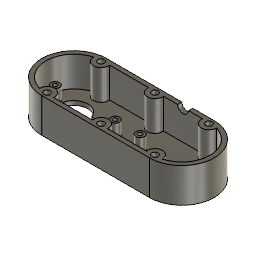
robosoc_motor_case_with_hole (Autodesk Fusion 360 design; units mm, degrees)
part number: 2025-12-10-15-49-31-313
Autodesk Fusion 360 part; units mm, degrees
sketch "Sketch1" plane through (0, 0, 0) normal (0, 0, 1) x (1, 0, 0)
  line L0 (15, 0) -> (65, 0)
  line L1 (65, 30) -> (15, 30)
  arc A0 (15, 30) -> (0, 15) centre (15, 15) ccw
  arc A1 (0, 15) -> (15, 0) centre (15, 15) ccw
  arc A2 (80, 15) -> (65, 30) centre (65, 15) ccw
  arc A3 (65, 0) -> (80, 15) centre (65, 15) ccw
  line L2 (15, 15) -> (65, 15) construction
  line L3 (15, 15) -> (15, 27.5) construction
  line L4 (65, 15) -> (65, 27.5) construction
  line L5 (15, 27.5) -> (40, 27.5) construction
  circle A4 centre (15, 27.5) radius 1.5
  circle A5 centre (40, 27.5) radius 1.5
  circle A6 centre (65, 27.5) radius 1.5
  circle A7 centre (15, 2.5) radius 1.5
  circle A8 centre (40, 2.5) radius 1.5
  circle A9 centre (65, 2.5) radius 1.5
  point P0 (80, 0)
  point P1 (0, 30)
  dimension "d1" = 80
  dimension "d2" = 30
  dimension "d3" = 15
  dimension "d4" = 15
  dimension "d5" = 15
  dimension "d6" = 15
  dimension "d7" = 12.5
  dimension "d8" = 12.5
  dimension "d9" = 25
  dimension "d11" = 3
  dimension "d12" = 3
  dimension "d13" = 3
  constraint horizontal L0
  constraint horizontal L1
  constraint coincident P1 L1
  constraint tangent L1 A0
  constraint coincident origin L0
  constraint tangent L0 A1
  constraint coincident A0.end A1.start
  constraint tangent L1 A2
  constraint coincident P0 L0
  constraint tangent L0 A3
  constraint coincident A2.start A3.end
  constraint coincident A0.centre A1.centre
  constraint coincident A2.centre A3.centre
  constraint perpendicular L1 L3
  constraint perpendicular L2 L4
  constraint perpendicular L3 L5
  constraint coincident L3.end L5.start
  constraint coincident L5.end A5.centre
  constraint coincident L4.end A6.centre
  constraint symmetric L2 A4 A7
  constraint symmetric L2 A5 A8
  constraint symmetric L2 A6 A9
  measures "d1" distance of origin P0
  measures "d2" distance of origin P1
  measures "d3" radius of A0
  measures "d4" radius of A1
  measures "d5" radius of A2
  measures "d6" radius of A3
  measures "d7" distance of A0.centre L3.end
  measures "d8" distance of A2.centre L4.end
  measures "d9" distance of L3.end L5.end
  measures "d11" diameter of A4
  measures "d12" diameter of A5
  measures "d13" diameter of A6
extrude "Extrude4" add sketch "Sketch1" along normal blind 2 contours A4 | A5 | A6 | A7 | A8 | A9 makes body 1 at (63.9526, 26.4262, 1.3333) makes body 2 at (41.4981, 2.4252, 1.3333) makes body 3 at (63.9526, 1.4262, 1.3333) makes body 4 at (38.9526, 26.4262, 1.3333) makes body 5 at (16.4981, 27.4252, 1.3333) makes body 6 at (16.4981, 2.4252, 1.3333)
extrude "Extrude1" add sketch "Sketch1" along normal blind 16 separate body makes body 7
shell "Shell1" thickness 2 removed faces 1 at (23.6999, 18.8266, 16) on bodies 7
sketch "Sketch2" plane through (0, 0, 2) normal (0, 0, 1) x (-1, 0, 0)
  arc A0 (-68.4999, -2.48) -> (-61.5359, -2) centre (-65, -2.5) ccw
  arc A1 (-68.4999, -2.48) -> (-68.4999, -27.52) centre (-65, -15) ccw
  arc A2 (-61.5359, -28) -> (-68.4999, -27.52) centre (-65, -27.5) ccw
  line L0 (-61.5359, -28) -> (-43.4641, -28)
  arc A3 (-36.5359, -28) -> (-43.4641, -28) centre (-40, -27.5) ccw
  line L1 (-36.5359, -28) -> (-18.4641, -28)
  arc A4 (-11.5001, -27.52) -> (-18.4641, -28) centre (-15, -27.5) ccw
  arc A5 (-11.5001, -27.52) -> (-11.5001, -2.48) centre (-15, -15) ccw
  arc A6 (-18.4641, -2) -> (-11.5001, -2.48) centre (-15, -2.5) ccw
  line L2 (-18.4641, -2) -> (-36.5359, -2)
  arc A7 (-43.4641, -2) -> (-36.5359, -2) centre (-40, -2.5) ccw
  line L3 (-43.4641, -2) -> (-61.5359, -2)
  line L4 (-15, -2.5) -> (-15, -27.5) construction
  arc A8 (-20.7264, -12.142) -> (-20.9934, -17.2449) centre (-21.0208, -14.6851) ccw
  arc A9 (-20.9934, -17.2449) -> (-20.7264, -12.142) centre (-15, -15) ccw
  arc A10 (-58.9129, -12.4127) -> (-58.8845, -17.522) centre (-64.7667, -15) ccw
  arc A11 (-58.8845, -17.522) -> (-58.9129, -12.4127) centre (-58.7336, -14.9664) ccw
  line L5 (-15, -15) -> (-34.1, -15) construction
  line L6 (-15, -15) -> (-6.3, -15) construction
  line L7 (-64.7667, -15) -> (-45.6667, -15) construction
  line L8 (-64.7667, -15) -> (-73.4667, -15) construction
  circle A12 centre (-6.3, -15) radius 1
  circle A13 centre (-34.1, -15) radius 1
  circle A14 centre (-73.4667, -15) radius 1
  circle A15 centre (-45.6667, -15) radius 1
  circle A16 centre (-34.1, -15) radius 2
  circle A17 centre (-6.3, -15) radius 2
  circle A18 centre (-45.6667, -15) radius 2
  circle A19 centre (-73.4667, -15) radius 2
  dimension "d17" = 12.8
  dimension "d18" = 12.8
  dimension "d19" = 5.12
  dimension "d20" = 5.12
  dimension "d22" = 19.1
  dimension "d23" = 8.7
  dimension "d24" = 19.1
  dimension "d25" = 8.7
  dimension "d26" = 2
  dimension "d27" = 2
  dimension "d29" = 2
  dimension "d31" = 2
  dimension "d32" = 1
  dimension "d33" = 1
  dimension "d34" = 1
  dimension "d35" = 1
  constraint coincident A6.centre L4.start
  constraint coincident A4.centre L4.end
  constraint concentric A5 A9
  constraint coincident A5.centre A9.centre
  constraint perpendicular L4 L5
  constraint perpendicular L4 L6
  constraint coincident A10.centre L7.start
  constraint parallel L1 L7
  constraint parallel L7 L8
  constraint coincident L6.end A12.centre
  constraint coincident L5.end A13.centre
  constraint coincident L8.end A14.centre
  constraint coincident L7.end A15.centre
  measures "d17" diameter of A9
  measures "d18" diameter of A10
  measures "d19" diameter of A8
  measures "d20" diameter of A11
  measures "d22" distance of A5.centre L5.end
  measures "d23" distance of A5.centre L6.end
  measures "d24" distance of A10.centre L7.end
  measures "d25" distance of A10.centre L8.end
  measures "d26" diameter of A12
  measures "d27" diameter of A13
  measures "d29" diameter of A14
  measures "d31" diameter of A15
  measures "d32" distance of A13
  measures "d33" distance of A12
  measures "d34" distance of A15
  measures "d35" distance of A14
extrude "Extrude2" cut sketch "Sketch2" against normal through all contours A8 A9 | A10 A11 bodies 7
extrude "Extrude3" add sketch "Sketch2" along normal blind 6.4 contours A16 | A17 | A18 | A19 bodies 7
sketch "Sketch3" plane through (0, 30, 0) normal (0, 1, 0) x (-1, 0, 0)
  line L0 (-65, 0) -> (-15, 0)
  line L1 (-15, 0) -> (-15, 16)
  line L2 (-15, 16) -> (-65, 16)
  line L3 (-65, 16) -> (-65, 0)
  line L4 (-65, 16) -> (-15, 16)
  line L5 (-65, 0) -> (-65, 16)
  line L6 (-65, 0) -> (-15, 0)
  line L7 (-15, 0) -> (-15, 16)
  line L8 (-65, 16) -> (-15, 16) construction
  line L9 (-65, 16) -> (-40, 16) construction
  line L10 (-65, 16) -> (-52.5, 16) construction
  circle A0 centre (-52.5, 16) radius 2.5
  dimension "d40" = 5
  constraint coincident L2.end L3.start
  constraint coincident L1.end L2.start
  constraint coincident L4 L9.end
  constraint midpoint L8 L9.end
  constraint midpoint L9 L10.end
  constraint coincident L10.end A0.centre
  measures "d40" diameter of A0
extrude "Extrude5" cut sketch "Sketch3" against normal up to surface (2 mm away) contours L2 L4 A0 picked at (-52.6854, 15.1876) bodies 7
equation "d3 = d4"
equation "d5 = d4"
equation "d6 = d4"
equation "d8 = d7"
equation "d11 = d12"
equation "d13 = d12"
equation "d17 = d18"
equation "d19 = d20"
equation "d20 = d18 / 2.5"
equation "d22 = d24"
equation "d23 = d25"
equation "d25 = 11 mm - 2.3 mm"
equation "d26 = d31"
equation "d27 = d31"
equation "d29 = d31"
equation "d32 = d34"
equation "d33 = d34"
equation "d35 = d34"
